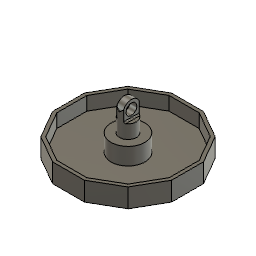
Calibration+Weight+Holder (Autodesk Fusion 360 design; units mm, degrees)
Autodesk Fusion 360 part; units mm, degrees
sketch "Sketch1" plane through (0, 0, 0) normal (0, 1, 0) x (1, 0, 0)
  circle A0 centre (0, 0) radius 24.875
  line L0 (-23.4897, 87.6649) -> (23.4897, 87.6649)
  line L1 (23.4897, 87.6649) -> (64.1752, 64.1752)
  line L2 (64.1752, 64.1752) -> (87.6649, 23.4897)
  line L3 (87.6649, 23.4897) -> (87.6649, -23.4897)
  line L4 (87.6649, -23.4897) -> (64.1752, -64.1752)
  line L5 (64.1752, -64.1752) -> (23.4897, -87.6649)
  line L6 (23.4897, -87.6649) -> (-23.4897, -87.6649)
  line L7 (-23.4897, -87.6649) -> (-64.1752, -64.1752)
  line L8 (-64.1752, -64.1752) -> (-87.6649, -23.4897)
  line L9 (-87.6649, -23.4897) -> (-87.6649, 23.4897)
  line L10 (-87.6649, 23.4897) -> (-64.1752, 64.1752)
  line L11 (-64.1752, 64.1752) -> (-23.4897, 87.6649)
  line L12 (-87.6649, 0) -> (0, 0) construction
  line L13 (0, 0) -> (87.6649, 0) construction
  line L14 (0, 0) -> (0, -87.6649) construction
  line L15 (0, 0) -> (0, 87.6649) construction
  line L16 (-22.15, 82.6649) -> (22.15, 82.6649)
  line L17 (22.15, 82.6649) -> (60.5149, 60.5149)
  line L18 (60.5149, 60.5149) -> (82.6649, 22.15)
  line L19 (82.6649, 22.15) -> (82.6649, -22.15)
  line L20 (82.6649, -22.15) -> (60.5149, -60.5149)
  line L21 (60.5149, -60.5149) -> (22.15, -82.6649)
  line L22 (22.15, -82.6649) -> (-22.15, -82.6649)
  line L23 (-22.15, -82.6649) -> (-60.5149, -60.5149)
  line L24 (-60.5149, -60.5149) -> (-82.6649, -22.15)
  line L25 (-82.6649, -22.15) -> (-82.6649, 22.15)
  line L26 (-82.6649, 22.15) -> (-60.5149, 60.5149)
  line L27 (-60.5149, 60.5149) -> (-22.15, 82.6649)
  line L28 (0, 0) -> (-82.6649, 0) construction
  line L29 (0, 0) -> (0, 82.6649) construction
  line L30 (0, 0) -> (82.6649, 0) construction
  line L31 (0, 0) -> (0, -82.6649) construction
  point P0 (24.875, 0)
  dimension "d1" = 49.75
  dimension "d3" = 150
  dimension "d4" = 62.7899
  dimension "d5" = 5
  dimension "d9" = 150
  dimension "d10" = 44.3
  constraint coincident A0.centre L12.end
  constraint horizontal L0
  constraint perpendicular L0 L3
  constraint perpendicular L3 L6
  constraint perpendicular L6 L9
  constraint midpoint L9 L12.start
  constraint midpoint L3 L13.end
  constraint midpoint L6 L14.end
  constraint midpoint L0 L15.end
  constraint equal L0 L1
  constraint equal L0 L2
  constraint equal L0 L3
  constraint equal L0 L4
  constraint equal L1 L5
  constraint equal L1 L6
  constraint equal L1 L7
  constraint equal L1 L8
  constraint equal L1 L9
  constraint equal L1 L10
  constraint equal L1 L11
  constraint horizontal L12
  constraint vertical L15
  constraint horizontal L13
  constraint vertical L14
  constraint equal L13 L15
  constraint equal L14 L15
  constraint equal L12 L15
  constraint coincident A0 P0
  constraint coincident L13 P0
  constraint perpendicular L15 L16
  constraint horizontal L22
  constraint perpendicular L12 L25
  constraint equal L16 L17
  constraint equal L17 L18
  constraint equal L18 L19
  constraint equal L19 L20
  constraint equal L20 L21
  constraint equal L21 L22
  constraint equal L22 L23
  constraint equal L23 L24
  constraint equal L24 L25
  constraint equal L25 L26
  constraint equal L26 L27
  constraint vertical L19
  constraint midpoint L25 L28.end
  constraint midpoint L16 L29.end
  constraint midpoint L19 L30.end
  constraint midpoint L22 L31.end
  constraint equal L28 L29
  constraint equal L29 L30
  constraint equal L29 L31
  constraint vertical L29
  constraint horizontal L30
  constraint horizontal L28
  constraint vertical L31
  measures "d1" diameter of A0
  measures "d3" angle of L0 L1
  measures "d4" distance of L3 P0
  measures "d5" distance of L0 L16
  measures "d9" angle of L16 L17
  measures "d10" distance of L16.start L16.end
extrude "Extrude1" add sketch "Sketch1" along normal blind 8 contours L16 L17 L18 L19 L20 L21 L22 L23 L24 L25 L26 L27
extrude "Extrude6" add sketch "Sketch1" along normal blind 28 contours L0 L1 L2 L3 L4 L5 L6 L7 L8 L9 L10 L11
extrude "Extrude2" add sketch "Sketch1" along normal blind 33 contours A0
sketch "Sketch2" plane through (0, 33, 0) normal (0, 1, 0) x (-1, 0, 0)
  circle A0 centre (0, 0) radius 24.875
  circle A1 centre (0, 0) radius 12.4375
  dimension "d15" = 49.75
  dimension "d16" = 24.875
  constraint coincident A0.centre A1.centre
  measures "d15" diameter of A0
  measures "d16" diameter of A1
extrude "Extrude3" add sketch "Sketch2" along normal blind 20 contours A1
sketch "Sketch3" plane through (0, 0, 0) normal (1, 0, 0) x (0, 0, -1)
  line L0 (12.4375, 53) -> (-12.4375, 53)
  line L1 (-12.4375, 33) -> (12.4375, 33)
  line L2 (0, 53) -> (0, 65.4375) construction
  circle A0 centre (0, 65.4375) radius 12.4375
  circle A1 centre (0, 65.4375) radius 8
  line L3 (0, 65.4375) -> (-12.4375, 65.4375) construction
  line L4 (0, 65.4375) -> (12.4375, 65.4375) construction
  line L5 (-12.4375, 65.4375) -> (-12.4375, 53)
  line L6 (12.4375, 65.4375) -> (12.4375, 53)
  dimension "d19" = 24.875
  dimension "d20" = 16
  dimension "d21" = 24.875
  constraint midpoint L0 L2.start
  constraint perpendicular L0 L2
  constraint coincident L2.end A0.centre
  constraint coincident L2.start A0
  constraint concentric A0 A1
  constraint coincident A0 L3.end
  constraint perpendicular L2 L3
  constraint coincident A0 L4.end
  constraint perpendicular L2 L4
  constraint coincident L0.end L5.end
  constraint coincident L0.start L6.end
  measures "d19" diameter of A0
  measures "d20" diameter of A1
  measures "d21" distance of L0.start L0.end
extrude "Extrude4" add sketch "Sketch3" along normal mid plane 10
extrude "Extrude5" cut 1 faces at (20.5903, 33, 1.8537) along direction (0, 1, 0) blind 50
fillet "Fillet1" radius 2 2 edges at (5, 53, 0) (-5, 53, 0)
sketch "Sketch4" plane through (0, 0, 0) normal (0, -1, 0) x (1, 0, 0)
  line L0 (-87.6649, -23.4897) -> (-64.1752, -64.1752)
  line L1 (-64.1752, -64.1752) -> (-23.4897, -87.6649)
  line L2 (-23.4897, -87.6649) -> (23.4897, -87.6649)
  line L3 (23.4897, -87.6649) -> (64.1752, -64.1752)
  line L4 (64.1752, -64.1752) -> (87.6649, -23.4897)
  line L5 (87.6649, -23.4897) -> (87.6649, 23.4897)
  line L6 (87.6649, 23.4897) -> (64.1752, 64.1752)
  line L7 (64.1752, 64.1752) -> (23.4897, 87.6649)
  line L8 (23.4897, 87.6649) -> (-23.4897, 87.6649)
  line L9 (-23.4897, 87.6649) -> (-64.1752, 64.1752)
  line L10 (-64.1752, 64.1752) -> (-87.6649, 23.4897)
  line L11 (-87.6649, 23.4897) -> (-87.6649, -23.4897)
  line L12 (0, 87.6649) -> (0, -87.6649) construction
  line L13 (87.6649, 0) -> (-87.6649, 0) construction
  circle A0 centre (0, 0) radius 13.725
  dimension "d30" = 27.45
  constraint midpoint L8 L12.start
  constraint midpoint L2 L12.end
  constraint midpoint L5 L13.start
  constraint midpoint L11 L13.end
  constraint coincident A0.centre origin
  measures "d30" diameter of A0
extrude "Extrude7" cut sketch "Sketch4" against normal blind 11 contours A0
equation "d9 = d3"
equation "d11 = 8 mm"
equation "d13 = d11 + 25 mm"
equation "d16 = d15 / 2"
equation "d19 = d21"
equation "d28 = d11 + 20 mm"
